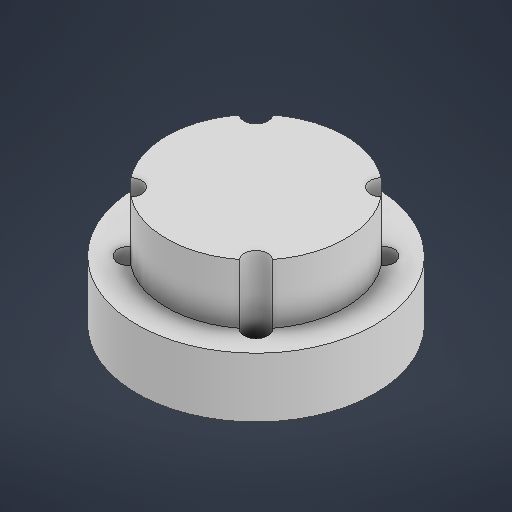
# Autodesk Inventor part: magnete
Saved by Autodesk Inventor 2027 (Build 310192060, 192F)
## iProperties
Created: 2026-07-02
Part Number: magnete
Material: Generic
Document SubType Name: Modeling
Designer: loren
Density: 1 g/cm^3
Appearance: Default
Author: loren
Autodesk Inventor part; units mm, degrees
ref_plane "YZ Plane" through (0, 0, 0) normal (1, 0, 0) x (0, 1, 0)
ref_plane "XZ Plane" through (0, 0, 0) normal (0, 1, 0) x (-1, 0, 0)
ref_plane "XY Plane" through (0, 0, 0) normal (0, 0, 1) x (1, 0, 0)
sketch "Sketch1" plane through (0, 0, 0) normal (0, 1, 0) x (-1, 0, 0)
  circle A0 centre (0, 0) radius 10
  circle A1 centre (0, 0) radius 7.5
  dimension "d0" = 20
  dimension "d1" = 15
  constraints: 2 centre point, 2 coincident
  measures "d0" diameter of A0
  measures "d1" diameter of A1
extrude "Extrusion1" add sketch "Sketch1" along normal blind 10 contours A1
extrude "Extrusion2" add sketch "Sketch1" along normal blind 5
sketch "Sketch2" plane through (0, 0, 0) normal (0, -1, 0) x (1, 0, 0)
  circle A0 centre (0, 0) radius 10 projected
  line L0 (0, 0) -> (10, 0) construction
  line L1 (7.0711, -7.0711) -> (6.0104, -6.0104)
  circle A1 centre (0, 0) radius 7.5 projected
  circle A2 centre (5.3033, 5.3033) radius 1
  line L2 (0, 0) -> (2.7588, 0)
  line L3 (0, 0) -> (0, -2.4662)
  circle A3 centre (5.3033, -5.3033) radius 1
  circle A4 centre (-5.3033, 5.3033) radius 1
  circle A5 centre (-5.3033, -5.3033) radius 1
  dimension "d7" = 2
  constraints: 8 end point, 3 centre point, 3 symmetric about line, 1 horizontal, 1 perpendicular, 1 point on line, 10 other
  measures "d7" diameter of A2
extrude "Extrusion3" cut sketch "Sketch2" against normal blind 10 contours A3 A1 | A3 A1 | A5 A1 | A1 A5 | A2 A1 | A1 A2 | A4 A1 | A1 A4
body "Solid1"
